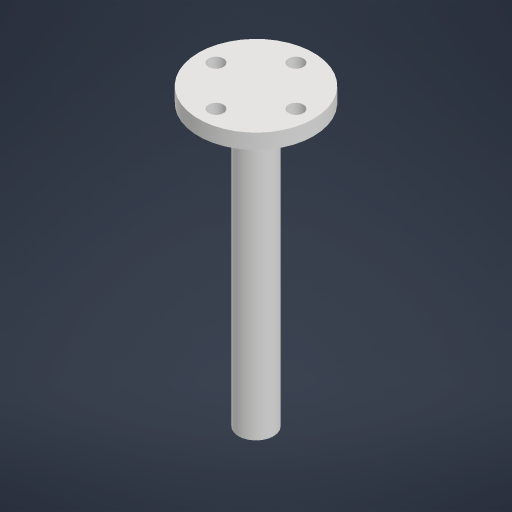
# Autodesk Inventor part: landing_gear
Saved by Autodesk Inventor 2024 (Build 280153000, 153)
## iProperties
Created: 2024-03-06
Part Number: landing_gear
Material: Generic
Document SubType Name: Modeling
Designer: skcre
Density: 1 g/cm^3
Appearance: Default
Author: skcre
Autodesk Inventor part; units mm, degrees
ref_plane "YZ Plane" through (0, 0, 0) normal (1, 0, 0) x (0, 1, 0)
ref_plane "XZ Plane" through (0, 0, 0) normal (0, 1, 0) x (-1, 0, 0)
ref_plane "XY Plane" through (0, 0, 0) normal (0, 0, 1) x (1, 0, 0)
sketch "Sketch1" plane through (0, 0, 0) normal (0, 1, 0) x (-1, 0, 0)
  circle A0 centre (0, 0) radius 11.5
  circle A1 centre (0, 0) radius 8
  circle A2 centre (0, -8) radius 1.5
  circle A3 centre (8, 0) radius 1.5
  circle A4 centre (0, 8) radius 1.5
  circle A5 centre (-8, 0) radius 1.5
  dimension "d0" = 23
  dimension "d1" = 16
  dimension "d2" = 3
  dimension "d3" = 3
  dimension "d4" = 3
  dimension "d5" = 3
  constraints: 6 centre point, 4 point on circle, 2 coincident
  measures "d0" diameter of A0
  measures "d1" diameter of A1
  measures "d2" diameter of A2
  measures "d3" diameter of A3
  measures "d4" diameter of A4
  measures "d5" diameter of A5
extrude "Extrusion1" add sketch "Sketch1" along normal blind 3 contours A0 | A3 A1 A2 A5 A4
sketch "Sketch2" plane through (0, 0, 0) normal (0, -1, 0) x (1, 0, 0)
  circle A0 centre (0, 0) radius 3.5
  dimension "d8" = 7
  constraints: 1 centre point, 1 coincident
  measures "d8" diameter of A0
extrude "Extrusion2" add sketch "Sketch2" along normal blind 56
fillet "Fillet2" radius 2 1 edges at (-3.5, 0, 0)
sketch "Sketch4" plane through (0, 0, 0) normal (0, -1, 0) x (1, 0, 0)
  circle A0 centre (0, 0) radius 3.5 projected
  circle A1 centre (0, 0) radius 11.5 projected
  circle A2 centre (8, 0) radius 1.5 projected
  circle A3 centre (0, -8) radius 1.5 projected
  circle A4 centre (-8, 0) radius 1.5 projected
  circle A5 centre (0, 8) radius 1.5 projected
body "Solid1"
